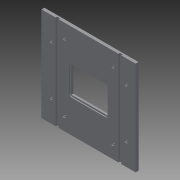
# Autodesk Inventor part: router_table_1
Saved by Autodesk Inventor 2013 (Build 170138000, 138)
## iProperties
Created: 2013-03-27
Part Number: router_table_1
Material: Generic
Document SubType Name: Modeling
Designer: TechShop Member
Density: 1 g/cm^3
Author: TechShop Member
Autodesk Inventor part; units mm, degrees
ref_plane "YZ Plane" through (0, 0, 0) normal (1, 0, 0) x (0, 1, 0)
ref_plane "XZ Plane" through (0, 0, 0) normal (0, 1, 0) x (-1, 0, 0)
ref_plane "XY Plane" through (0, 0, 0) normal (0, 0, 1) x (1, 0, 0)
sketch "Sketch1" plane through (0, 0, 0) normal (0, 0, 1) x (1, 0, 0)
  line L0 (-304.6106, 302.7116) -> (304.9894, 302.7116)
  line L1 (304.9894, 302.7116) -> (304.9894, -306.8884)
  line L2 (304.9894, -306.8884) -> (-304.6106, -306.8884)
  line L3 (-304.6106, -306.8884) -> (-304.6106, 302.7116)
  point P0 (0, 0)
  dimension "d0" = 609.6
  dimension "d2" = 609.6
  constraints: 8 end point, 2 parallel, 1 horizontal, 1 perpendicular
  measures "d0" distance of L2.end L0.start
  measures "d2" distance of L0.end L0.start
extrude "Extrusion1" add sketch "Sketch1" along normal blind 19.05
sketch "Sketch2" plane through (0, 0, 19.05) normal (0, 0, 1) x (1, 0, 0)
  circle A0 centre (-242.6981, -160.8384) radius 4.7625
  circle A1 centre (243.0642, -160.8384) radius 4.7625
  circle A2 centre (243.0642, 156.6616) radius 4.7625
  circle A3 centre (-242.6981, 156.6616) radius 4.7625
  circle A4 centre (-157.7669, -219.5759) radius 4.7625
  circle A5 centre (158.1456, -219.5759) radius 4.7625
  circle A6 centre (158.1456, 215.3991) radius 4.7625
  circle A7 centre (-157.7669, 215.3991) radius 4.7625
  point P0 (-304.6106, -306.8884)
  point P1 (0, 0)
  point P2 (304.9894, 302.7116)
  point P3 (-304.6106, 302.7116)
  point P4 (304.9894, -306.8884)
  dimension "d5" = 9.525
  dimension "d6" = 146.05
  dimension "d7" = 61.9125
  dimension "d15" = 9.525
  dimension "d16" = 146.05
  dimension "d17" = 61.9252
  dimension "d18" = 9.525
  dimension "d19" = 61.9252
  dimension "d20" = 146.05
  dimension "d21" = 9.525
  dimension "d22" = 61.9125
  dimension "d23" = 146.05
  dimension "d24" = 9.525
  dimension "d25" = 146.8438
  dimension "d26" = 87.3125
  dimension "d27" = 9.525
  dimension "d28" = 146.8438
  dimension "d29" = 87.3125
  dimension "d30" = 9.525
  dimension "d31" = 87.3125
  dimension "d32" = 146.8438
  dimension "d33" = 9.525
  dimension "d34" = 146.8438
  dimension "d35" = 87.3125
  constraints: 8 centre point
  measures "d5" diameter of A0
  measures "d6" vertical distance of point (-304.611, -306.888) A0.centre
  measures "d7" horizontal distance of point (-304.611, -306.888) A0.centre
  measures "d15" diameter of A1
  measures "d16" vertical distance of point (304.989, -306.888) A1.centre
  measures "d17" horizontal distance of point (304.989, -306.888) A1.centre
  measures "d18" diameter of A2
  measures "d19" horizontal distance of point (304.989, 302.712) A2.centre
  measures "d20" vertical distance of point (304.989, 302.712) A2.centre
  measures "d21" diameter of A3
  measures "d22" horizontal distance of point (-304.611, 302.712) A3.centre
  measures "d23" vertical distance of point (-304.611, 302.712) A3.centre
  measures "d24" diameter of A4
  measures "d25" horizontal distance of point (-304.611, -306.888) A4.centre
  measures "d26" vertical distance of point (-304.611, -306.888) A4.centre
  measures "d27" diameter of A5
  measures "d28" horizontal distance of A5.centre point (304.989, -306.888)
  measures "d29" vertical distance of point (304.989, -306.888) A5.centre
  measures "d30" diameter of A6
  measures "d31" vertical distance of point (304.989, 302.712) A6.centre
  measures "d32" horizontal distance of point (304.989, 302.712) A6.centre
  measures "d33" diameter of A7
  measures "d34" horizontal distance of point (-304.611, 302.712) A7.centre
  measures "d35" vertical distance of point (-304.611, 302.712) A7.centre
hole "Hole2" at (-242.6981, -160.8384, 19.05) at (-242.6981, 156.6616, 19.05) at (-157.7669, 215.3991, 19.05) at (158.1456, 215.3991, 19.05) at (243.0642, 156.6616, 19.05) at (243.0642, -160.8384, 19.05) at (158.1456, -219.5759, 19.05) at (-157.7669, -219.5759, 19.05) direction (0, 0, -1) diameter 9.525 end through all counterbore diameter 25.4 counterbore depth 4.7625
sketch "Sketch3" plane through (0, 0, 19.05) normal (0, 0, 1) x (1, 0, 0)
  line L0 (-117.475, -85.725) -> (117.475, -85.725)
  line L1 (117.475, -85.725) -> (117.475, 85.725)
  line L2 (117.475, 85.725) -> (-117.475, 85.725)
  line L3 (-117.475, 85.725) -> (-117.475, -85.725)
  line L4 (-117.475, -85.725) -> (117.475, 85.725) construction
  line L5 (117.475, -85.725) -> (-117.475, 85.725) construction
  point P0 (0, 0)
  dimension "d43" = 234.95
  dimension "d44" = 171.45
  constraints: 12 end point, 2 midpoint, 2 parallel, 1 horizontal, 1 perpendicular
  measures "d43" distance of L2.end L1.end
  measures "d44" distance of L1.end L0.end
extrude "Extrusion2" cut sketch "Sketch3" against normal blind 19.05
sketch "Sketch4" plane through (0, 0, 19.05) normal (0, 0, 1) x (1, 0, 0)
  line L0 (117.475, 85.725) -> (117.475, -85.725) projected
  line L1 (117.475, -85.725) -> (-117.475, -85.725) projected
  line L2 (-117.475, -85.725) -> (-117.475, 85.725) projected
  line L3 (-117.475, 85.725) -> (117.475, 85.725) projected
  arc A0 (-107.95, 95.25) -> (-127, 76.2) centre (-107.95, 76.2) ccw
  line L4 (-107.95, 76.2) -> (-107.95, 95.25) construction
  line L5 (-107.95, 76.2) -> (-88.9, 76.2) construction
  line L6 (-107.95, 76.2) -> (-127, 76.2) construction
  arc A1 (-127, -80.1017) -> (-108.2751, -95.25) centre (-108.2751, -76.1028) ccw
  arc A2 (108.1693, -95.25) -> (127, -75.9762) centre (107.9478, -76.1978) ccw
  line L7 (107.9478, -76.1978) -> (127, -75.9762) construction
  line L8 (107.9478, -76.1978) -> (108.1693, -95.25) construction
  arc A3 (127, 76.5685) -> (108.3185, 95.25) centre (108.3185, 76.5685) ccw
  line L9 (127, -75.9762) -> (127, 76.5685)
  line L10 (-107.95, 95.25) -> (108.3185, 95.25)
  line L11 (108.1693, -95.25) -> (-108.2751, -95.25)
  line L12 (-127, 76.2) -> (-127, -80.1017)
  point P0 (0, 0)
  dimension "d47" = 19.05
  dimension "d48" = 90
  dimension "d49" = 90
  dimension "d50" = 9.525
  dimension "d51" = 9.525
  dimension "d52" = 9.525
  dimension "d53" = 9.525
  dimension "d54" = 90
  dimension "d55" = 9.525
  dimension "d56" = 9.525
  dimension "d57" = 9.525
  dimension "d58" = 9.525
  constraints: 18 end point, 8 point on circle, 4 centre point, 4 tangent, 3 perpendicular, 1 horizontal, 1 parallel
  measures "d47" radius of A0
  measures "d48" angle of L5 L4
  measures "d49" angle of L4 L6
  measures "d50" horizontal distance of L4.end L2.end
  measures "d51" horizontal distance of L6.end L2.end
  measures "d52" horizontal distance of L12.end L1.end
  measures "d53" vertical distance of L11.end L1.end
  measures "d54" angle of L8 L7
  measures "d55" vertical distance of L0.end L8.end
  measures "d56" horizontal distance of L7.end L0.end
  measures "d57" horizontal distance of L9.end L0.start
  measures "d58" vertical distance of L0.start L10.end
extrude "Extrusion3" cut sketch "Sketch4" against normal blind 6.35
sketch "Sketch5" plane through (0, 0, 19.05) normal (0, 0, 1) x (1, 0, 0)
  line L0 (-304.6106, 302.7116) -> (-304.6106, -306.8884) projected
  line L1 (-304.6106, -306.8884) -> (304.9894, -306.8884) projected
  line L2 (304.9894, -306.8884) -> (304.9894, 302.7116) projected
  line L3 (-212.5356, 306.8884) -> (-193.4856, 306.8884)
  line L4 (-193.4856, 306.8884) -> (-193.4856, -306.8884)
  line L5 (-193.4856, -306.8884) -> (-212.5356, -306.8884)
  line L6 (-212.5356, -306.8884) -> (-212.5356, 306.8884)
  line L7 (-212.5356, 306.8884) -> (-193.4856, -306.8884) construction
  line L8 (-193.4856, 306.8884) -> (-212.5356, -306.8884) construction
  line L9 (193.8644, 306.8884) -> (212.9144, 306.8884)
  line L10 (212.9144, 306.8884) -> (212.9144, -306.8884)
  line L11 (212.9144, -306.8884) -> (193.8644, -306.8884)
  line L12 (193.8644, -306.8884) -> (193.8644, 306.8884)
  line L13 (193.8644, 306.8884) -> (212.9144, -306.8884) construction
  line L14 (212.9144, 306.8884) -> (193.8644, -306.8884) construction
  point P0 (0, 0)
  point P1 (-203.0106, 0)
  point P2 (203.3894, 0)
  dimension "d61" = 19.05
  dimension "d62" = 101.6
  dimension "d63" = 19.05
  dimension "d64" = 101.6
  constraints: 24 end point, 4 midpoint, 4 parallel, 2 horizontal, 2 perpendicular, 2 point on line
  measures "d61" distance of L4.end L5.end
  measures "d62" distance from line of L0 point (-203.011, 0)
  measures "d63" distance of L10.end L11.end
  measures "d64" distance from line of L2 point (203.389, 0)
extrude "Extrusion4" cut sketch "Sketch5" against normal blind 9.525
body "Solid1"
